Autodesk Inventor part; units mm, degrees
(part 2 of 2)
extrude "Extrusion7" add sketch "Sketch10" along normal blind 0.1 contours L8 S0 L9 S1 L10 L11 L12 S2 S3 L13 L14 | L18 S6 L19 L20 S7 L21 L22 L23 L24 L25 L26 L27 L28 L29 L30 L31 L32 L33 L34 S8 L35 L36 S9 L37 L38 L39 L40 | L41 L42 L43 S10 L44 L45 L46 L47 L48 S11 L49 S12 L50 L51 L52 L53 L54 L55 L56 S13 L57 L58 L59 L60 L61 S14 L62 L63 L64 L65 | L66 S15 L67 L68 L69 L70 S16 L71 L72 L73 L74 L75 L76 L77 L78 L79 L80 L81 L82 | L88 S17 L89 S18 L90 L91 L92 L93 L94 L95 L96 L97 L98 L99 S19 L100 S20 L101 L102 L103 L104 L105 S21 L106 L107 L108 L109 L110 L111 L112 L113 L114 L115 S22 L116 L117 L118 L119 | L120 S23 L121 S24 L122 L123 L124 L125 L126 S25 L127 S26 L128 L129 L130 L131 | L132 S27 L133 L134 S28 L135 L136 L137 L138 L139 L140 L141 L142 L143 L144 L145 L146 L147 L148 S29 L149 L150 S30 L151 L152 L153 L154 L155 L156 L157 L158 L159 L160 L161 L162 L163 | L164 S31 L165 S32 L166 L167 L168 L169 L170 L171 S33 L172 L173 L174 S34 L175 L176 L177 L178 L179 S35 L180 L181 L182 S36 L183 L184 L185 L186 L187 | L188 S37 L189 S38 L190 L191 L192 L193 L194 S39 L195 L196 S40 L197 L198 L199 L200 L201 | L202 L203 S41 S42 L204 L205 L206 L207 L208 S43 S44 L209 S45 S46 L210 L211 L212 L213 L214 L215 L216 S47 S48 L217 S49 S50 L218 L219 L220 L221 L222 S51 S52 L223 L224 L225 | L226 S53 L227 L228 L229 S54 S55 S56 S57 L230 L231 S58 S59 L232 L233 L234 S60 S61 L235 L236 S62 L237 L238 L239 S63 S64 L240 L241 S65 S66 S67 L242 L243 L244 S68 S69 L245 | L246 L247 L248 L249 | L250 S70 S71 S72 S73 S74 S75 S76 S77 L251 | L252 L253 L254 L255 L256 L257 L258 L259 L260 L261 L262
body "Solid1"
